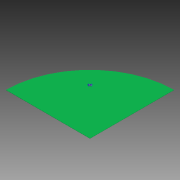
# Autodesk Inventor part: top-wafer
Saved by Autodesk Inventor 2011 SP1 (Build 150282100, 282)
## iProperties
Created: 2011-03-24
Part Number: top-wafer
Document SubType Name: Modeling
Designer: Andrew Zonenberg
Density: 1 g/cm^3
Author: Andrew Zonenberg
Autodesk Inventor part; units mm, degrees
ref_plane "YZ Plane" through (0, 0, 0) normal (1, 0, 0) x (0, 1, 0)
ref_plane "XZ Plane" through (0, 0, 0) normal (0, 1, 0) x (-1, 0, 0)
ref_plane "XY Plane" through (0, 0, 0) normal (0, 0, 1) x (1, 0, 0)
sketch "Sketch1" plane through (0, 0, 0) normal (0, 0, 1) x (1, 0, 0)
  line L0 (0, 0) -> (-50, 0)
  line L1 (0, 0) -> (0, 50)
  arc A0 (0, 50) -> (-50, 0) centre (0, 0) ccw
  dimension "d0" = 50
  constraints: 4 end point, 2 perpendicular, 2 point on circle, 1 centre point, 1 coincident, 1 horizontal
  measures "d0" distance of L0.start L0.end
extrude "Wafer" add sketch "Sketch1" along normal blind 0.1
fillet "OuterEdge" radius 0.1 1 edges at (-35.3553, 35.3553, 0)
sketch "DeepEtchSketch" plane through (0, 0, 0.1) normal (0, 0, 1) x (1, 0, 0)
  line L0 (0, 0) -> (-50, 0) projected
  line L1 (0, 50) -> (0, 0) projected
  line L2 (-25, 25) -> (-15, 25) construction
  line L3 (-15, 25) -> (-15, 15) construction
  line L4 (-15, 15) -> (-25, 15) construction
  line L5 (-25, 15) -> (-25, 25) construction
  line L6 (-25, 20) -> (-15, 20) construction
  line L7 (-20, 25) -> (-20, 15) construction
  line L8 (-27.875, 27.875) -> (-27.125, 27.875) construction
  line L9 (-27.125, 27.875) -> (-27.125, 27.125) construction
  line L10 (-27.125, 27.125) -> (-27.875, 27.125) construction
  line L11 (-27.875, 27.125) -> (-27.875, 27.875) construction
  line L12 (-27.875, 27.875) -> (-28.625, 27.875)
  line L13 (-28.625, 27.875) -> (-28.625, 27.125)
  line L14 (-28.625, 27.125) -> (-27.875, 27.125)
  line L15 (-27.875, 27.125) -> (-27.875, 26.375)
  line L16 (-27.875, 26.375) -> (-27.125, 26.375)
  line L17 (-27.125, 26.375) -> (-27.125, 27.125)
  line L18 (-27.875, 27.875) -> (-27.875, 28.625)
  line L19 (-27.875, 28.625) -> (-27.125, 28.625)
  line L20 (-27.125, 28.625) -> (-27.125, 27.875)
  line L21 (-26.375, 27.875) -> (-27.125, 27.875)
  line L22 (-26.375, 27.875) -> (-26.375, 27.125)
  line L23 (-26.375, 27.125) -> (-27.125, 27.125)
  line L24 (-27.875, 27.5) -> (-27.125, 27.5) construction
  line L25 (-27.5, 27.875) -> (-27.5, 27.125) construction
  dimension "d4" = 20
  dimension "d5" = 20
  dimension "d6" = 10
  dimension "d7" = 0.75
  dimension "d12" = 2.5
  dimension "d13" = 2.5
  constraints: 48 end point, 16 perpendicular, 8 midpoint, 8 parallel, 2 horizontal
  measures "d4" distance between parallel lines of L1 L7
  measures "d5" distance between parallel lines of L0 L6
  measures "d6" distance between parallel lines of L3 L5
  measures "d7" distance between parallel lines of L10 L8
  measures "d12" distance between parallel lines of L2 L24
  measures "d13" distance between parallel lines of L5 L25
extrude "ThroughWaferEtch" cut sketch "DeepEtchSketch" against normal blind 0.1 draft -57.6
body "Solid1"
